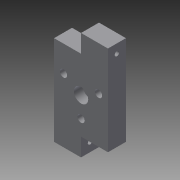
# Autodesk Inventor part: MotorMount
Saved by Autodesk Inventor 2013 (Build 170138000, 138)
## iProperties
Created: 2013-10-23
Part Number: MotorMount
Material: Generic
Document SubType Name: Modeling
Designer: cobrooks
Density: 1 g/cm^3
Author: cobrooks
Autodesk Inventor part; units mm, degrees
ref_plane "YZ Plane" through (0, 0, 0) normal (1, 0, 0) x (0, 1, 0)
ref_plane "XZ Plane" through (0, 0, 0) normal (0, 1, 0) x (-1, 0, 0)
ref_plane "XY Plane" through (0, 0, 0) normal (0, 0, 1) x (1, 0, 0)
sketch "Sketch1" plane through (0, 0, 0) normal (0, 0, 1) x (1, 0, 0)
  line L0 (-19.05, -38.1) -> (19.05, -38.1)
  line L1 (19.05, -38.1) -> (19.05, 38.1)
  line L2 (19.05, 38.1) -> (-19.05, 38.1)
  line L3 (-19.05, 38.1) -> (-19.05, -38.1)
  line L4 (-19.05, -38.1) -> (19.05, 38.1) construction
  line L5 (19.05, -38.1) -> (-19.05, 38.1) construction
  point P0 (0, 0)
  dimension "d0" = 38.1
  dimension "d1" = 76.2
  constraints: 12 end point, 2 midpoint, 2 parallel, 1 horizontal, 1 perpendicular
  measures "d0" distance of L2.end L1.end
  measures "d1" distance of L1.end L0.end
extrude "Extrusion1" add sketch "Sketch1" along normal blind 12.7
sketch "Sketch2" plane through (0, 0, 12.7) normal (0, 0, 1) x (1, 0, 0)
  line L0 (-19.05, 38.1) -> (0, 38.1)
  line L1 (0, 38.1) -> (0, 25.4)
  line L2 (0, 25.4) -> (-19.05, 25.4)
  line L3 (-19.05, 25.4) -> (-19.05, 38.1)
  point P0 (0, 0)
  dimension "d4" = 19.05
  dimension "d5" = 12.7
  constraints: 8 end point, 2 parallel, 1 horizontal, 1 perpendicular
  measures "d4" distance of L1.end L2.end
  measures "d5" distance of L0.end L1.end
extrude "Extrusion2" cut sketch "Sketch2" against normal blind 12.7
sketch "Sketch3" plane through (0, 0, 12.7) normal (0, 0, 1) x (1, 0, 0)
  line L0 (19.05, -38.1) -> (0, -38.1)
  line L1 (0, -38.1) -> (0, -25.4)
  line L2 (0, -25.4) -> (19.05, -25.4)
  line L3 (19.05, -25.4) -> (19.05, -38.1)
  point P0 (0, 0)
  dimension "d8" = 19.05
  dimension "d9" = 12.7
  constraints: 8 end point, 2 parallel, 1 horizontal, 1 perpendicular
  measures "d8" distance of L1.end L2.end
  measures "d9" distance of L0.end L1.end
extrude "Extrusion3" cut sketch "Sketch3" against normal blind 12.7
sketch "Sketch4" plane through (0, 0, 12.7) normal (0, 0, 1) x (1, 0, 0)
  circle A0 centre (0, 0) radius 5.08
  dimension "d12" = 10.16
  constraints: 1 centre point, 1 coincident
  measures "d12" diameter of A0
extrude "Extrusion4" cut sketch "Sketch4" against normal blind 6.35
sketch "Sketch5" plane through (19.05, 38.1, 12.7) normal (1, 0, 0) x (0, 0, -1)
  line L0 (12.7, -76.2) -> (12.7, 0) projected
  line L1 (12.7, 0) -> (0, 0) projected
  line L2 (0, -63.5) -> (0, 0) projected
  line L3 (0, -12.7) -> (12.7, -12.7) projected
  circle A0 centre (6.35, -6.35) radius 1.5875
  point P0 (12.7, -63.5)
  point P1 (12.7, -38.1)
  dimension "d16" = 3.175
  dimension "d17" = 6.35
  dimension "d18" = 6.35
  dimension "d19" = 6.35
  dimension "d20" = 6.35
  constraints: 1 centre point
  measures "d16" diameter of A0
  measures "d17" distance from line of L0 A0.centre
  measures "d18" distance from line of L2 A0.centre
  measures "d19" distance from line of L3 A0.centre
  measures "d20" distance from line of L1 A0.centre
extrude "Extrusion5" cut sketch "Sketch5" against normal blind 19.05 contours A0
sketch "Sketch7" plane through (0, 0, 12.7) normal (0, 0, 1) x (1, 0, 0)
  circle A0 centre (12.3917, 7.1543) radius 2.54 projected
  circle A1 centre (-12.3917, 7.1543) radius 2.54 projected
  circle A2 centre (0, -14.3087) radius 2.54 projected
extrude "Extrusion7" cut sketch "Sketch7" against normal blind 6.35
sketch "Sketch9" plane through (-19.05, -38.1, 0) normal (-1, 0, 0) x (0, 0, 1)
  line L0 (0, 0) -> (12.7, 0) projected
  line L1 (12.7, 63.5) -> (12.7, 0) projected
  line L2 (12.7, 12.5394) -> (0, 12.5394) projected
  circle A0 centre (6.35, 6.2697) radius 1.5875
  point P0 (0, 38.1)
  dimension "d34" = 3.175
  dimension "d35" = 6.35
  dimension "d36" = 6.2697
  dimension "d37" = 6.2697
  constraints: 1 centre point
  measures "d34" diameter of A0
  measures "d35" distance from line of L1 A0.centre
  measures "d36" distance from line of L0 A0.centre
  measures "d37" distance from line of L2 A0.centre
extrude "Extrusion9" cut sketch "Sketch9" against normal blind 19.05
equation "\"d17\" = d18"
equation "\"d19\" = d20"
equation "\"d36\" = d37"
body "Solid1"
